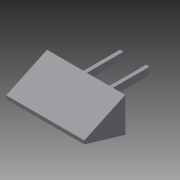
# Autodesk Inventor part: Prow
Saved by Autodesk Inventor 2015 (Build 190159000, 159)
## iProperties
Created: 2016-01-19
Part Number: Prow
Material: Generic
Document SubType Name: Modeling
Designer: sethbattis
Density: 1 g/cm^3
Appearance: Default
Author: sethbattis
Autodesk Inventor part; units mm, degrees
ref_plane "YZ Plane" through (0, 0, 0) normal (1, 0, 0) x (0, 1, 0)
ref_plane "XZ Plane" through (0, 0, 0) normal (0, 1, 0) x (-1, 0, 0)
ref_plane "XY Plane" through (0, 0, 0) normal (0, 0, 1) x (1, 0, 0)
sketch "Sketch1" plane through (0, 0, 0) normal (1, 0, 0) x (0, 1, 0)
  line L0 (-127, 35.9623) -> (-127, -77.6639) construction
  line L1 (0, -169.3966) -> (0, 472.7328) construction
  line L2 (-202.8496, 0) -> (248.9132, 0) construction
  line L3 (76.331, 381) -> (-138.3121, 381) construction
  line L4 (177.8, 0) -> (50.8, 0) construction
  line L5 (50.8, 0) -> (50.8, 50.8) construction
  line L6 (82.55, 82.55) -> (146.05, 82.55) construction
  line L7 (177.8, 50.8) -> (177.8, 0) construction
  arc A0 (177.8, 50.8) -> (146.05, 82.55) centre (146.05, 50.8) ccw construction
  arc A1 (82.55, 82.55) -> (50.8, 50.8) centre (82.55, 50.8) ccw construction
  line L8 (0, 381) -> (-25.4, 381)
  line L9 (-25.4, 381) -> (-113.2817, 82.55)
  line L10 (-113.2817, 82.55) -> (139.2767, 82.55)
  line L11 (0, 381) -> (177.8, 0) construction
  line L12 (139.2767, 82.55) -> (0, 381)
  line L13 (-25.4, 381) -> (-127, 35.9623) construction
  point P0 (0, 0)
  point P1 (50.8, 82.55)
  point P2 (177.8, 82.55)
  dimension "d2" = 127
  dimension "d3" = 381
  dimension "d4" = 127
  dimension "d5" = 82.55
  dimension "d6" = 304.8
  dimension "d7" = 31.75
  dimension "d8" = 25.4
  constraints: 24 end point, 9 point on line, 4 point on circle, 4 tangent, 3 collinear, 2 centre point, 2 horizontal, 2 parallel, 1 equal radius, 1 perpendicular, 1 vertical
  measures "d2" distance between parallel lines of L0 L1
  measures "d3" distance between parallel lines of L3 L2
  measures "d4" distance of point (50.8, 82.55) point (177.8, 82.55)
  measures "d5" distance of L4.end point (50.8, 82.55)
  measures "d6" distance between parallel lines of L0 L7
  measures "d7" radius of A0
  measures "d8" distance of L8.start L8.end
extrude "Extrusion1" add sketch "Sketch1" along normal blind 571.5
sketch "Sketch2" plane through (0, -113.2817, 82.55) normal (0, 0, -1) x (-1, 0, 0)
  line L0 (0, 0) -> (0, 252.5584) construction
  line L1 (0, 252.5584) -> (-571.5, 252.5584) construction
  line L2 (-571.5, 0) -> (-571.5, 252.5584) construction
  line L3 (0, 0) -> (-571.5, 0) construction
  line L4 (-393.7, 164.0817) -> (-368.3, 164.0817)
  line L5 (-368.3, 164.0817) -> (-368.3, 113.2817)
  line L6 (-368.3, 113.2817) -> (-393.7, 113.2817)
  line L7 (-393.7, 113.2817) -> (-393.7, 164.0817)
  line L8 (0, 113.2817) -> (-571.5, 113.2817) projected
  line L9 (-203.2, 164.0817) -> (-177.8, 164.0817)
  line L10 (-177.8, 164.0817) -> (-177.8, 113.2817)
  line L11 (-177.8, 113.2817) -> (-203.2, 113.2817)
  line L12 (-203.2, 113.2817) -> (-203.2, 164.0817)
  line L13 (0, 252.5584) -> (-571.5, 252.5584) construction
  line L14 (-285.75, 252.5584) -> (-285.75, 0) construction
  dimension "d29" = 25.4
  dimension "d30" = 50.8
  dimension "d31" = 215.9
  constraints: 18 end point, 4 parallel, 2 equal length, 2 horizontal, 2 midpoint, 2 perpendicular, 2 point on line, 1 other
  measures "d29" distance of L5.end L6.end
  measures "d30" distance of L4.end L5.end
  measures "d31" distance between parallel lines of L10 L7
extrude "Extrusion2" add sketch "Sketch2" along normal blind 355.6
body "Solid1"
